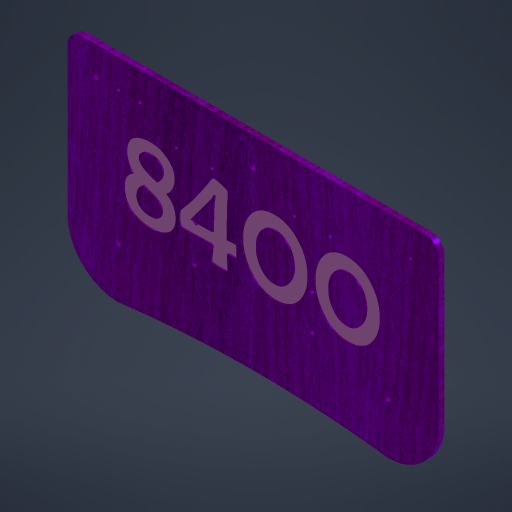
# Autodesk Inventor part: FTC Outside Panels
Saved by Autodesk Inventor 2024.2 (Build 282272000, 272)
## iProperties
Created: 2022-09-22
Part Number: FTC Outside Panels
Material: Wood (Oak)
Document SubType Name: Modeling
Designer: Jason
Density: 0.76 g/cm^3
Appearance: Birch - Natural Polished
Mass: 371.39 g
Surface Area: 1832.51 cm^2
Volume: 488.671 cm^3
Author: Allan
Autodesk Inventor part; units mm, degrees
ref_plane "YZ Plane" through (0, 0, 0) normal (1, 0, 0) x (0, 1, 0)
ref_plane "XZ Plane" through (0, 0, 0) normal (0, 1, 0) x (-1, 0, 0)
ref_plane "XY Plane" through (0, 0, 0) normal (0, 0, 1) x (1, 0, 0)
sketch "Sketch1" plane through (0, 0, 0) normal (0, 0, 1) x (1, 0, 0)
  line L0 (0, 0) -> (333.375, 0)
  line L1 (333.375, 0) -> (333.375, 177.8)
  line L2 (320.675, 190.5) -> (12.7, 190.5)
  line L3 (0, 177.8) -> (0, 0)
  circle A0 centre (45.72, 45.72) radius 45.72
  circle A1 centre (287.655, 45.72) radius 45.72
  line L4 (166.6875, 0) -> (166.6875, 7.62)
  arc A2 (287.655, 0) -> (45.72, 0) centre (166.6875, -956.3695) ccw
  arc A3 (12.7, 190.5) -> (0, 177.8) centre (12.7, 177.8) ccw
  arc A4 (333.375, 177.8) -> (320.675, 190.5) centre (320.675, 177.8) ccw
  circle A5 centre (45.72, 45.72) radius 2.413
  circle A6 centre (287.655, 45.72) radius 2.413
  circle A7 centre (25.4, 165.1) radius 2.413
  circle A8 centre (307.975, 165.1) radius 1.2446
  line L5 (25.4, 165.1) -> (307.975, 165.1)
  circle A9 centre (166.6875, 165.1) radius 2.413
  ellipse E0 centre (219.583, 63.3371) end of major axis (219.5756, 65.3371) minor radius 2
  line L6 (219.583, 45.72) -> (219.583, 63.3371)
  ellipse E1 centre (113.792, 63.3371) end of major axis (113.7846, 65.3371) minor radius 2
  line L7 (113.792, 45.72) -> (113.792, 63.3371)
  circle A10 centre (219.583, 79.3382) radius 4.699
  circle A11 centre (113.792, 79.3371) radius 4.699
  line L8 (219.583, 95.3392) -> (219.583, 63.3371)
  line L9 (113.792, 95.337) -> (113.792, 63.3371)
  line L10 (45.72, 45.72) -> (113.792, 45.72)
  line L11 (287.655, 45.72) -> (219.583, 45.72)
  ellipse E2 centre (219.583, 95.3392) end of major axis (219.5791, 97.3392) minor radius 2
  ellipse E3 centre (113.792, 95.337) end of major axis (113.7881, 97.337) minor radius 2
  point P0 (333.375, 190.5)
  point P1 (0, 190.5)
  point P2 (0, 45.72)
  point P3 (333.375, 45.72)
  dimension "d79" = 91.44
  dimension "d80" = 91.44
  dimension "d77" = 333.375
  dimension "d78" = 190.5
  dimension "d81" = 7.62
  dimension "d82" = 12.7
  dimension "d84" = 4.826
  dimension "d85" = 4.826
  dimension "d86" = 4.826
  dimension "d87" = 25.4
  dimension "d88" = 25.4
  dimension "d90" = 2.4892
  dimension "d91" = 25.4
  dimension "d92" = 25.4
  dimension "d94" = 4.826
  dimension "d95" = 17.6171
  dimension "d97" = 17.6171
  dimension "d98" = 9.398
  dimension "d99" = 9.398
  dimension "d103" = 68.072
  dimension "d104" = 68.072
  dimension "d114" = 32.0021
  dimension "d115" = 31.9999
  constraints: 24 end point, 10 centre point, 7 point on circle, 6 coincident, 6 point on line, 6 vertical, 5 horizontal, 4 midpoint, 4 tangent, 2 parallel, 1 equal radius, 1 perpendicular, 14 other
  measures "d77" distance of point (0, 190.5) point (333.375, 190.5)
  measures "d78" distance of point (333.375, 190.5) L0.end
  measures "d81" distance of L4.start L4.end
  measures "d82" radius of A3
  measures "d84" diameter of A5
  measures "d85" diameter of A6
  measures "d86" diameter of A7
  measures "d87" distance from line of L2 L5.start
  measures "d88" distance from line of L3 L5.start
  measures "d90" diameter of A8
  measures "d91" distance from line of L1 L5.end
  measures "d92" distance from line of L2 L5.end
  measures "d94" diameter of A9
  measures "d95" distance of L6.start L6.end
  measures "d97" distance of L7.start L9.end
  measures "d98" diameter of A10
  measures "d99" diameter of A11
  measures "d103" distance of L10.start L7.start
  measures "d104" distance of L11.start L6.start
  measures "d114" distance of L6.end L8.start
  measures "d115" distance of point (113.792, 63.337) point (113.792, 95.337)
extrude "Extrusion1" add sketch "Sketch1" along normal blind 5.08 contours A0 A2 | L3 A3 L2 A4 L1 A1 A2 A0 | A2 A1 | A10 L8 | L8 A10 | A11 L9 | L9 A11 picked at (30.9641, 18.3065) picked at (302.4109, 18.3065)
sketch "Sketch9" plane through (0, 0, 5.08) normal (0, 0, 1) x (1, 0, 0)
  line L0 (25.0687, 165.288) -> (307.7817, 165.288) construction
  line L1 (307.7817, 165.288) -> (307.7817, 45.2815) construction
  line L2 (307.7817, 45.2815) -> (25.0687, 45.2815) construction
  line L3 (25.0687, 45.2815) -> (25.0687, 165.288) construction
  spline S0 degree 2 poles (97.0599, 90.5973) (97.0599, 81.7558) (90.2543, 76.4625) knots 0 0 0 1 1 1
  spline S1 degree 2 poles (90.2543, 76.4625) (83.9721, 71.4601) (74.3744, 71.4601) knots 0 0 0 1 1 1
  spline S2 degree 2 poles (74.3744, 71.4601) (63.7297, 71.4601) (57.5057, 76.0554) knots 0 0 0 1 1 1
  spline S3 degree 2 poles (57.5057, 76.0554) (50.2347, 81.4068) (50.2347, 91.9934) knots 0 0 0 1 1 1
  spline S4 degree 2 poles (50.2347, 91.9934) (50.2347, 101.6493) (58.4946, 106.3027) knots 0 0 0 1 1 1
  spline S5 degree 2 poles (58.4946, 106.3027) (55.7607, 108.3967) (52.3869, 116.3076) (52.3869, 120.3212) knots 0 0 0 1 2 2 2
  spline S6 degree 2 poles (52.3869, 120.3212) (52.3869, 129.3372) (59.1926, 134.3396) knots 0 0 0 1 1 1
  spline S7 degree 2 poles (59.1926, 134.3396) (65.3002, 138.8186) (74.5489, 138.8186) knots 0 0 0 1 1 1
  spline S8 degree 2 poles (74.5489, 138.8186) (82.9833, 138.8186) (89.2072, 133.9906) knots 0 0 0 1 1 1
  spline S9 degree 2 poles (89.2072, 133.9906) (96.1292, 128.8137) (96.1292, 120.6702) knots 0 0 0 1 1 1
  spline S10 degree 2 poles (96.1292, 120.6702) (96.1292, 116.5403) (94.0352, 112.3522) knots 0 0 0 1 1 1
  spline S11 degree 2 poles (94.0352, 112.3522) (91.9993, 107.9896) (88.5674, 105.721) knots 0 0 0 1 1 1
  spline S12 degree 2 poles (88.5674, 105.721) (97.0599, 100.8349) (97.0599, 90.5973) knots 0 0 0 1 1 1
  spline S13 degree 2 poles (84.3793, 89.8412) (84.3793, 94.6691) (78.039, 97.8102) knots 0 0 0 1 1 1
  spline S14 degree 2 poles (78.039, 97.8102) (72.8621, 99.7879) (67.6851, 101.7656) knots 0 0 0 1 1 1
  spline S15 degree 2 poles (67.6851, 101.7656) (61.8683, 97.8102) (61.8683, 91.2954) knots 0 0 0 1 1 1
  spline S16 degree 2 poles (61.8683, 91.2954) (61.8683, 86.8746) (64.8349, 84.0825) knots 0 0 0 1 1 1
  spline S17 degree 2 poles (64.8349, 84.0825) (68.0923, 81.0578) (73.9672, 81.0578) knots 0 0 0 1 1 1
  spline S18 degree 2 poles (73.9672, 81.0578) (84.3793, 81.0578) (84.3793, 89.8412) knots 0 0 0 1 1 1
  spline S19 degree 2 poles (85.2518, 120.0303) (85.2518, 123.6949) (79.2605, 128.9882) (74.8979, 128.9882) knots 0 0 0 1 2 2 2
  spline S20 degree 2 poles (74.8979, 128.9882) (69.8373, 128.9882) (64.0205, 124.9746) (64.0205, 121.7172) knots 0 0 0 1 2 2 2
  spline S21 degree 2 poles (64.0205, 121.7172) (64.0205, 117.5291) (70.1282, 114.3299) knots 0 0 0 1 1 1
  spline S22 degree 2 poles (70.1282, 114.3299) (72.8621, 112.8757) (80.4239, 110.4326) knots 0 0 0 1 1 1
  spline S23 degree 2 poles (80.4239, 110.4326) (85.2518, 114.4462) (85.2518, 120.0303) knots 0 0 0 1 1 1
  spline S24 degree 2 poles (151.5633, 87.5144) (151.5633, 86.4674) (150.3999, 86.5256) knots 0 0 0 1 1 1
  spline S25 degree 2 poles (150.3999, 86.5256) (148.4804, 86.6419) (144.9903, 86.6419) knots 0 0 0 1 1 1
  spline S26 degree 2 poles (144.9903, 86.6419) (143.7106, 86.6419) (143.4779, 86.4674) knots 0 0 0 1 1 1
  spline S27 degree 2 poles (143.4779, 86.4674) (143.0708, 86.2348) (143.0708, 85.0132) knots 0 0 0 1 1 1
  spline S28 degree 2 poles (143.0708, 85.0132) (143.0708, 83.1519) (143.6524, 75.6482) (143.6524, 73.7868) knots 0 0 0 1 2 2 2
  spline S29 degree 2 poles (143.6524, 73.7868) (143.6524, 72.6235) (142.3146, 72.3908) knots 0 0 0 1 1 1
  spline S30 degree 2 poles (142.3146, 72.3908) (140.5114, 72.0999) (136.1488, 72.0999) knots 0 0 0 1 1 1
  spline S31 degree 2 poles (136.1488, 72.0999) (128.7033, 72.0999) (128.7033, 73.2633) knots 0 0 0 1 1 1
  spline S32 degree 2 poles (128.7033, 73.2633) (128.7033, 74.8338) (129.8666, 83.3845) (129.8666, 85.4204) knots 0 0 0 1 2 2 2
  spline S33 degree 2 poles (129.8666, 85.4204) (129.8666, 86.6419) (128.936, 86.6419) knots 0 0 0 1 1 1
  spline S34 degree 2 poles (128.936, 86.6419) (124.6315, 86.6419) (107.472, 86.1184) (103.1676, 86.1184) knots 0 0 0 1 2 2 2
  spline S35 degree 2 poles (103.1676, 86.1184) (99.9683, 86.1184) (99.9683, 92.6332) knots 0 0 0 1 1 1
  spline S36 degree 2 poles (99.9683, 92.6332) (99.9683, 97.8102) (101.0153, 99.0317) knots 0 0 0 1 1 1
  spline S37 degree 2 poles (101.0153, 99.0317) (104.6799, 103.2198) (111.5437, 111.8868) knots 0 0 0 1 1 1
  spline S38 degree 2 poles (111.5437, 111.8868) (120.0944, 123.8694) (124.806, 131.0241) knots 0 0 0 1 1 1
  spline S39 degree 2 poles (124.806, 131.0241) (126.3184, 133.3508) (129.4013, 137.9461) knots 0 0 0 1 1 1
  spline S40 degree 2 poles (129.4013, 137.9461) (130.2738, 139.1094) (131.03, 139.1094) knots 0 0 0 1 1 1
  spline S41 degree 2 poles (131.03, 139.1094) (134.6946, 139.1094) (142.2564, 136.3755) knots 0 0 0 1 1 1
  spline S42 degree 2 poles (142.2564, 136.3755) (143.8851, 135.7938) (143.8851, 134.3978) knots 0 0 0 1 1 1
  spline S43 degree 2 poles (143.8851, 134.3978) (143.8851, 131.7221) (143.0708, 120.7865) (143.0708, 118.1108) knots 0 0 0 1 2 2 2
  spline S44 degree 2 poles (143.0708, 118.1108) (143.0708, 115.6677) (143.0126, 109.6764) knots 0 0 0 1 1 1
  spline S45 degree 2 poles (143.0126, 109.6764) (142.8963, 104.325) (142.9544, 101.3003) knots 0 0 0 1 1 1
  line L4 (142.9544, 101.3003) -> (142.9544, 96.9958)
  spline S46 degree 2 poles (142.9544, 96.9958) (144.3505, 96.9958) (149.7019, 97.403) (151.0398, 97.403) knots 0 0 0 1 2 2 2
  spline S47 degree 2 poles (151.0398, 97.403) (151.4469, 97.403) (151.4469, 96.5305) knots 0 0 0 1 1 1
  spline S48 degree 2 poles (151.4469, 96.5305) (151.4469, 95.0181) (151.5633, 89.0268) (151.5633, 87.5144) knots 0 0 0 1 2 2 2
  spline S49 degree 2 poles (131.7862, 125.3818) (131.7862, 125.789) (131.4953, 126.0216) knots 0 0 0 1 1 1
  spline S50 degree 2 poles (131.4953, 126.0216) (130.9718, 126.0216) (130.0993, 124.2184) knots 0 0 0 1 1 1
  spline S51 degree 2 poles (130.0993, 124.2184) (129.5758, 122.9969) (128.9941, 121.8917) knots 0 0 0 1 1 1
  spline S52 degree 2 poles (128.9941, 121.8917) (119.7454, 109.5601) (110.5549, 97.054) knots 0 0 0 1 1 1
  spline S53 degree 2 poles (110.5549, 97.054) (110.8457, 96.4723) (114.8593, 96.4723) knots 0 0 0 1 1 1
  line L5 (114.8593, 96.4723) -> (117.0115, 96.4723)
  spline S54 degree 2 poles (117.0115, 96.4723) (125.9112, 96.4723) (130.2738, 96.7632) knots 0 0 0 1 1 1
  spline S55 degree 2 poles (130.2738, 96.7632) (130.332, 103.278) (130.4483, 109.7928) knots 0 0 0 1 1 1
  spline S56 degree 2 poles (130.4483, 109.7928) (130.681, 118.1108) (131.379, 122.5315) knots 0 0 0 1 1 1
  spline S57 degree 2 poles (131.379, 122.5315) (131.7862, 125.0909) (131.7862, 125.3818) knots 0 0 0 1 1 1
  spline S58 degree 2 poles (215.4317, 104.9648) (215.4317, 91.5862) (207.5208, 81.9303) knots 0 0 0 1 1 1
  spline S59 degree 2 poles (207.5208, 81.9303) (199.0865, 71.5764) (185.9405, 71.5764) knots 0 0 0 1 1 1
  spline S60 degree 2 poles (185.9405, 71.5764) (172.8527, 71.5764) (164.4184, 81.9303) knots 0 0 0 1 1 1
  spline S61 degree 2 poles (164.4184, 81.9303) (156.4494, 91.6444) (156.4494, 104.9648) knots 0 0 0 1 1 1
  spline S62 degree 2 poles (156.4494, 104.9648) (156.4494, 118.3435) (164.4184, 127.9412) knots 0 0 0 1 1 1
  spline S63 degree 2 poles (164.4184, 127.9412) (172.8527, 138.1787) (185.9405, 138.1787) knots 0 0 0 1 1 1
  spline S64 degree 2 poles (185.9405, 138.1787) (199.0865, 138.1787) (207.5208, 127.9993) knots 0 0 0 1 1 1
  spline S65 degree 2 poles (207.5208, 127.9993) (215.4317, 118.3435) (215.4317, 104.9648) knots 0 0 0 1 1 1
  spline S66 degree 2 poles (202.9256, 104.9648) (202.9256, 113.1665) (198.6211, 119.1578) knots 0 0 0 1 1 1
  spline S67 degree 2 poles (198.6211, 119.1578) (193.8514, 125.6726) (185.9405, 125.6726) knots 0 0 0 1 1 1
  spline S68 degree 2 poles (185.9405, 125.6726) (178.0297, 125.6726) (173.2599, 119.1578) knots 0 0 0 1 1 1
  spline S69 degree 2 poles (173.2599, 119.1578) (169.0718, 113.2828) (169.0718, 104.9648) knots 0 0 0 1 1 1
  spline S70 degree 2 poles (169.0718, 104.9648) (169.0718, 96.8213) (173.3181, 90.7719) knots 0 0 0 1 1 1
  spline S71 degree 2 poles (173.3181, 90.7719) (178.0879, 84.0825) (185.9405, 84.0825) knots 0 0 0 1 1 1
  spline S72 degree 2 poles (185.9405, 84.0825) (193.4442, 84.0825) (198.4466, 90.9464) knots 0 0 0 1 1 1
  spline S73 degree 2 poles (198.4466, 90.9464) (202.9256, 97.1703) (202.9256, 104.9648) knots 0 0 0 1 1 1
  spline S74 degree 2 poles (280.4053, 104.9648) (280.4053, 91.5862) (272.4944, 81.9303) knots 0 0 0 1 1 1
  spline S75 degree 2 poles (272.4944, 81.9303) (264.0601, 71.5764) (250.9141, 71.5764) knots 0 0 0 1 1 1
  spline S76 degree 2 poles (250.9141, 71.5764) (237.8263, 71.5764) (229.392, 81.9303) knots 0 0 0 1 1 1
  spline S77 degree 2 poles (229.392, 81.9303) (221.423, 91.6444) (221.423, 104.9648) knots 0 0 0 1 1 1
  spline S78 degree 2 poles (221.423, 104.9648) (221.423, 118.3435) (229.392, 127.9412) knots 0 0 0 1 1 1
  spline S79 degree 2 poles (229.392, 127.9412) (237.8263, 138.1787) (250.9141, 138.1787) knots 0 0 0 1 1 1
  spline S80 degree 2 poles (250.9141, 138.1787) (264.0601, 138.1787) (272.4944, 127.9993) knots 0 0 0 1 1 1
  spline S81 degree 2 poles (272.4944, 127.9993) (280.4053, 118.3435) (280.4053, 104.9648) knots 0 0 0 1 1 1
  spline S82 degree 2 poles (267.8992, 104.9648) (267.8992, 113.1665) (263.5947, 119.1578) knots 0 0 0 1 1 1
  spline S83 degree 2 poles (263.5947, 119.1578) (258.825, 125.6726) (250.9141, 125.6726) knots 0 0 0 1 1 1
  spline S84 degree 2 poles (250.9141, 125.6726) (243.0033, 125.6726) (238.2335, 119.1578) knots 0 0 0 1 1 1
  spline S85 degree 2 poles (238.2335, 119.1578) (234.0454, 113.2828) (234.0454, 104.9648) knots 0 0 0 1 1 1
  spline S86 degree 2 poles (234.0454, 104.9648) (234.0454, 96.8213) (238.2917, 90.7719) knots 0 0 0 1 1 1
  spline S87 degree 2 poles (238.2917, 90.7719) (243.0614, 84.0825) (250.9141, 84.0825) knots 0 0 0 1 1 1
  spline S88 degree 2 poles (250.9141, 84.0825) (258.4178, 84.0825) (263.4202, 90.9464) knots 0 0 0 1 1 1
  spline S89 degree 2 poles (263.4202, 90.9464) (267.8992, 97.1703) (267.8992, 104.9648) knots 0 0 0 1 1 1
  point P0 (0, 0)
  dimension "d78" = 190.5
  constraints: 2 other
extrude "Extrusion9" cut sketch "Sketch9" against normal blind 1.27
sketch "Sketch10" plane through (0, 0, 5.08) normal (0, 0, 1) x (1, 0, 0)
  ellipse E0 centre (235.5574, 128.7087) end of major axis (235.5548, 130.0613) minor radius 1.3525 projected
  circle A0 centre (203.6555, 146.1392) radius 1.3589
  circle A1 centre (235.6554, 146.1392) radius 1.3589
  circle A2 centre (166.6875, 165.1) radius 2.413 projected
  line L0 (166.6875, 165.1) -> (166.6875, 65.684)
  circle A3 centre (129.7195, 146.1392) radius 1.3589
  circle A4 centre (97.7196, 146.1392) radius 1.3589
  ellipse E1 centre (219.583, 95.3392) end of major axis (219.5869, 93.3392) minor radius 2 projected
  line L1 (219.583, 146.1392) -> (235.6554, 146.1392)
  line L2 (235.6554, 146.1392) -> (203.6555, 146.1392)
  line L3 (219.583, 146.1392) -> (219.583, 95.3392)
  line L4 (203.6555, 146.1392) -> (97.7196, 146.1392)
  ellipse E2 centre (113.792, 95.337) end of major axis (113.7959, 93.337) minor radius 2 (115.4386, 96.4723) -> (112.2157, 96.568) ccw projected
  line L5 (219.583, 95.3392) -> (113.792, 95.337)
  point P0 (0, 0)
  point P1 (97.8176, 128.7087)
  dimension "d119" = 2.7178
  dimension "d120" = 2.7178
  dimension "d131" = 50.8
  dimension "d132" = 90.001
  constraints: 12 end point, 4 centre point, 3 symmetric about line, 2 horizontal, 2 vertical, 1 coincident, 1 collinear, 4 other
  measures "d119" diameter of A0
  measures "d120" diameter of A1
  measures "d131" distance of L1.start L3.end
  measures "d132" angle of L5 L0
extrude "Extrusion10" cut sketch "Sketch10" against normal blind 25.4 contours L2 L4 A0 | A0 L4 L2 | A1 | L4 A3 | A3 L4 | A4
sketch "Sketch12" plane through (0, 0, 5.08) normal (0, 0, 1) x (1, 0, 0)
  circle A0 centre (25.4, 165.1) radius 2.413 projected
  line L0 (27.813, 165.1) -> (25.4, 165.1)
  line L1 (25.4, 165.1) -> (45.847, 165.1)
  circle A1 centre (45.847, 165.1) radius 1.3589
  line L2 (45.847, 165.1) -> (64.897, 165.1)
  circle A2 centre (64.897, 165.1) radius 1.3589
  point P0 (0, 0)
  dimension "d124" = 20.447
  dimension "d125" = 2.7178
  dimension "d126" = 19.05
  dimension "d127" = 2.7178
  constraints: 6 end point, 2 centre point, 2 coincident, 2 horizontal, 1 horizontal alignment, 1 point on line, 1 other
  measures "d124" distance of L0.end L1.end
  measures "d125" diameter of A1
  measures "d126" distance of L2.start L2.end
  measures "d127" diameter of A2
extrude "Extrusion11" cut sketch "Sketch12" against normal blind 31.75 contours A1 L2 L1 | L1 L2 A1 | A2
body "Solid1"
